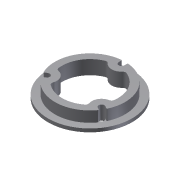
# Autodesk Inventor part: JointB0_
Saved by Autodesk Inventor 2011 SP1 (Build 150282100, 282)
## iProperties
Created: 2012-10-27
Part Number: JointB0_
Document SubType Name: Modeling
Designer: arihon
Density: 1 g/cm^3
Author: arihon
Autodesk Inventor part; units mm, degrees
ref_plane "YZ Plane" through (0, 0, 0) normal (1, 0, 0) x (0, 1, 0)
ref_plane "XZ Plane" through (0, 0, 0) normal (0, 1, 0) x (-1, 0, 0)
ref_plane "XY Plane" through (0, 0, 0) normal (0, 0, 1) x (1, 0, 0)
sketch "スケッチ1" plane through (0, 0, 0) normal (0, 0, 1) x (1, 0, 0)
  circle A0 centre (0, 0) radius 25
  dimension "d0" = 50
  constraints: 1 centre point, 1 coincident
  measures "d0" diameter of A0
extrude "押し出し1" add sketch "スケッチ1" along normal blind 7.6
sketch "スケッチ2" plane through (0, 0, 0) normal (0, 0, -1) x (-1, 0, 0)
  circle A0 centre (0, 0) radius 25 projected
  circle A1 centre (0, 0) radius 30
  dimension "d3" = 60
  constraints: 1 centre point, 1 coincident
  measures "d3" diameter of A1
extrude "押し出し2" add sketch "スケッチ2" along normal blind 2.4 contours A0 | A1
sketch "スケッチ3" plane through (0, 0, 7.6) normal (0, 0, 1) x (1, 0, 0)
  circle A0 centre (0, 0) radius 25 projected
  line L0 (0, 0) -> (0, 25)
  line L1 (0, 0) -> (21.6506, -12.5)
  line L2 (0, 0) -> (-21.6506, -12.5)
  circle A1 centre (0, 0) radius 22.5
  point P0 (0, 22.5)
  point P1 (19.4856, -11.25)
  point P2 (-19.4856, -11.25)
  dimension "d6" = 120
  dimension "d7" = 120
  dimension "d8" = 45
  constraints: 6 end point, 6 point on circle, 3 point on line, 1 centre point, 1 coincident, 1 vertical
  measures "d6" angle of L1 L0
  measures "d7" angle of L2 L1
  measures "d8" diameter of A1
hole "Hole1" at (0, 22.5, 7.6) at (19.4856, -11.25, 7.6) at (-19.4856, -11.25, 7.6) direction (0, 0, -1) diameter 4 end through all
shell "シェル1" thickness 5 removed faces 1 at (0, 0.0908, 7.6)
sketch "スケッチ4" plane through (0, 0, 7.6) normal (0, 0, 1) x (1, 0, 0)
  arc A0 (19.5432, -4.2502) -> (6.0908, 19.05) centre (0, 0) ccw projected
  arc A1 (-13.4524, -14.7998) -> (13.4524, -14.7998) centre (0, 0) ccw projected
  circle A2 centre (0, 22.5) radius 2 projected
  circle A3 centre (0, 0) radius 25 projected
  line L0 (-2, 22.5) -> (2, 22.5)
  line L1 (2, 22.5) -> (2, 25)
  line L2 (2, 25) -> (-2, 25)
  line L3 (-2, 25) -> (-2, 22.5)
  line L4 (-18.4856, -12.9821) -> (-20.4856, -9.5179)
  line L5 (-20.4856, -9.5179) -> (-22.6506, -10.7679)
  line L6 (-22.6506, -10.7679) -> (-20.6506, -14.2321)
  line L7 (-20.6506, -14.2321) -> (-18.4856, -12.9821)
  line L8 (20.4856, -9.5179) -> (18.4856, -12.9821)
  line L9 (18.4856, -12.9821) -> (20.6506, -14.2321)
  line L10 (20.6506, -14.2321) -> (22.6506, -10.7679)
  line L11 (22.6506, -10.7679) -> (20.4856, -9.5179)
  dimension "d17" = 4
  dimension "d18" = 2.5
  dimension "d21" = 360
  constraints: 24 end point, 2 parallel, 1 horizontal, 1 horizontal alignment, 1 perpendicular, 32 other
  measures "d17" distance of L0.start L0.end
  measures "d18" distance of L0.end L1.end
extrude "押し出し3" cut sketch "スケッチ4" against normal up to surface (7.6 mm away) contours L0 A2 | A2 L3 A3 L1 | A3 L2 L1 | L3 L2 A3 | L5 L4 L7 A3 | A3 L6 L5 | L11 L10 A3 | A3 L9 L8 L11 | A3 L7 L6 | L10 L9 A3 picked at (0.2364, 23.1233)
sketch "スケッチ5" plane through (0, 0, 2.6) normal (0, 0, 1) x (1, 0, 0)
  arc A0 (-13.4524, -14.7998) -> (13.4524, -14.7998) centre (0, 0) ccw projected
  arc A1 (19.5432, -4.2502) -> (13.4524, -14.7998) centre (19.4856, -11.25) ccw projected
  arc A2 (19.5432, -4.2502) -> (6.0908, 19.05) centre (0, 0) ccw projected
  arc A3 (-6.0908, 19.05) -> (6.0908, 19.05) centre (0, 22.5) ccw projected
  arc A4 (-6.0908, 19.05) -> (-19.5432, -4.2502) centre (0, 0) ccw projected
  arc A5 (-13.4524, -14.7998) -> (-19.5432, -4.2502) centre (-19.4856, -11.25) ccw projected
extrude "押し出し4" cut sketch "スケッチ5" against normal through all
fillet "フィレット1" radius 2 12 edges at (-6.0908, 19.05, 5.1) (-6.0908, 19.05, 0.1) (6.0908, 19.05, 5.1) (6.0908, 19.05, 0.1) (19.5432, -4.2502, 5.1) (19.5432, -4.2502, 0.1) (13.4524, -14.7998, 5.1) (13.4524, -14.7998, 0.1) (-13.4524, -14.7998, 5.1) (-13.4524, -14.7998, 0.1) (-19.5432, -4.2502, 5.1) (-19.5432, -4.2502, 0.1)
fillet "フィレット2" radius 0.5 6 edges at (2, 24.9199, 3.8) (-2, 24.9199, 3.8) (-22.5812, -10.7279, 3.8) (-20.5812, -14.192, 3.8) (20.5812, -14.192, 3.8) (22.5812, -10.7279, 3.8)
